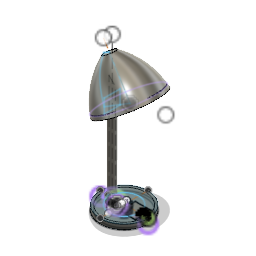
snailed_it v20 (Autodesk Fusion 360 design; units mm, degrees)
Autodesk Fusion 360 part; units mm, degrees
note: some values were not read from the file. Chosen so that the rebuilt part matches the saved one: which bodies a step acts on; a direction; which face or edge a step refers to. Set by a fixed rule: which sketch regions a step uses.
sketch "Sketch1" plane through (0, 0, 0) normal (0, 1, 0) x (1, 0, 0)
  circle A0 centre (0, 0) radius 150
  circle A1 centre (0, 0) radius 135
  dimension "d1" = 300
  dimension "d2" = 270
  constraint coincident A0.centre A1.centre
  measures "d1" diameter of A0
  measures "d2" diameter of A1
extrude "Extrude1" add sketch "Sketch1" along normal blind 30 makes body 1
sketch "Sketch2" plane through (0, 30, 0) normal (0, 1, 0) x (-1, 0, 0)
  circle A0 centre (0, 0) radius 135
  circle A1 centre (0, 0) radius 150
extrude "Extrude2" add sketch "Sketch2" along normal blind 2 separate body contours A0 | A1 makes body 2
sketch "Sketch3" plane through (0, 32, 0) normal (0, 1, 0) x (-1, 0, 0)
  circle A0 centre (0, 0) radius 150
  line L0 (0, 150) -> (0, 100) construction
  line L1 (0, 50) -> (0, -150) construction
  line L2 (150, 0) -> (-150, 0) construction
  circle A1 centre (75, 0) radius 25
  circle A2 centre (75, 0) radius 24
  point P0 (100, 0)
  point P1 (50, 0)
  dimension "d100" = 50
  dimension "d101" = 48
  dimension "d102" = 50
  dimension "d103" = 200
  constraint coincident A0 L0.start
  constraint coincident A0 L1.end
  constraint vertical L1
  constraint coincident A0 L2.start
  constraint coincident A0 L2.end
  constraint perpendicular L1 L2
  constraint coincident L2 A1.centre
  constraint concentric A1 A2
  constraint coincident L2 P0
  constraint coincident A1 P0
  constraint coincident A1 P1
  constraint coincident L2 P1
  measures "d100" diameter of A1
  measures "d101" diameter of A2
  measures "d102" distance of L2.start P0
  measures "d103" distance of L2.end P1
sketch "Sketch25" plane through (0, 0, 0) normal (0, 1, 0) x (1, 0, 0)
  circle A0 centre (-75, 0) radius 15
  point P0 (-75, 0)
  dimension "d142" = 30
  constraint coincident P0 A0.centre
  measures "d142" diameter of A0
extrude "Extrude4" cut sketch "Sketch25" along normal blind 130 bodies 2
extrude "Extrude3" add sketch "Sketch3" along normal blind 10 separate body contours A1 makes body 3
sketch "Sketch4" plane through (0, 32, 0) normal (0, 1, 0) x (-1, 0, 0)
  circle A0 centre (75, 0) radius 24
  circle A1 centre (75, 0) radius 23
  dimension "d104" = 48
  dimension "d105" = 46
  constraint concentric A0 A1
  measures "d104" diameter of A0
  measures "d105" diameter of A1
extrude "Extrude5" add sketch "Sketch4" along normal blind 700 separate body makes body 4
sketch "Sketch5" plane through (0, 30, 0) normal (0, 1, 0) x (-1, 0, 0)
  circle A0 centre (0, 0) radius 40
  circle A1 centre (0, 0) radius 91.8342
  dimension "d17" = 80
  constraint coincident A0.centre A1.centre
  constraint concentric A0 A1
  measures "d17" diameter of A0
sketch "Sketch6" plane through (0, 0, 0) normal (0, 0, 1) x (1, 0, 0)
  line L0 (150, 0) -> (-150, 0)
  line L1 (-75, 0) -> (0, 0) construction
  line L2 (-75, 0) -> (-75, 918.0902) construction
  line L3 (-55, 0) -> (-55, 645) construction
  line L4 (-95, 0) -> (-95, 685) construction
  line L5 (-95, 685) -> (-55, 645) construction
  point P0 (-75, 0)
  dimension "d106" = 75
  dimension "d108" = 20
  dimension "d109" = 20
  dimension "d110" = 685
  dimension "d112" = 45
  constraint perpendicular L1 L2
  constraint coincident L1.end origin
  constraint coincident L1 L3.start
  constraint coincident L0 L3.start
  constraint perpendicular L1 L3
  constraint coincident L0 L4.start
  constraint perpendicular L0 L4
  constraint coincident P0 L1.start
  measures "d106" distance of L1.end L1.start
  measures "d108" distance of L3.start P0
  measures "d109" distance of L4.start P0
  measures "d110" distance of L4.start L4.end
  measures "d112" angle of L4 L5
ref_plane "WorkPlane1" through (-75, 665, 0) normal (-0.707107, -0.707107, 0) x (0.707107, -0.707107, 0)
split "Split1" by plane through (-75, 665, 0) normal (-0.707107, -0.707107, 0) bodies 4 makes body 5 at (-66.9562, 448.9028, 22.6119)
delete_body "RemoveBody1" bodies 4
sketch "Sketch7" plane through (295, 295, 0) normal (-0.707107, -0.707107, 0) x (0.707107, -0.707107, 0)
  circle A0 centre (-523.2616, 0) radius 61
  point P0 (-523.2616, 0)
  dimension "d113" = 122
  constraint coincident P0 A0.centre
  measures "d113" diameter of A0
extrude "Extrude8" add sketch "Sketch7" against normal blind 2 separate body makes body 6
sketch "Sketch8" plane through (296.4142, 296.4142, 0) normal (0.707107, 0.707107, 0) x (0, 0, -1)
  circle A0 centre (0, 523.2616) radius 51
  circle A1 centre (0, 523.2616) radius 61
  point P0 (0, 523.2616)
  point P1 (0.1543, 462.2618)
  dimension "d32" = 102
  constraint coincident P0 A0.centre
  constraint coincident A1 P1
  measures "d32" diameter of A0
extrude "Extrude9" add sketch "Sketch8" along normal blind 6 separate body contours A0 makes body 7
sketch "Sketch9" plane through (296.4142, 296.4142, 0) normal (0.707107, 0.707107, 0) x (0, 0, -1)
  circle A0 centre (0, 523.2616) radius 61
  circle A1 centre (0, 523.2616) radius 52
  circle A2 centre (0, 523.2616) radius 61
  line L0 (-26.4064, 478.4654) -> (-31.9044, 471.2701)
  line L1 (26.4064, 478.4654) -> (31.9044, 471.2701)
  point P0 (0, 523.2616)
  dimension "d35" = 122
  dimension "d36" = 104
  constraint concentric A0 A1
  constraint coincident P0 A0.centre
  constraint coincident A1 L0.start
  constraint coincident A2 L0.end
  constraint coincident A1 L1.start
  constraint coincident A2 L1.end
  constraint coincident A0 L1.end
  constraint equal L0 L1
  measures "d35" diameter of A0
  measures "d36" diameter of A1
extrude "Extrude10" add sketch "Sketch9" along normal blind 6 separate body contours A0 A1 A2 L0 L1 picked at (-34.6439, 476.9097) makes body 8
sketch "Sketch10" plane through (300.6569, 300.6569, 0) normal (0.707107, 0.707107, 0) x (0, 0, -1)
  circle A0 centre (0, 523.2616) radius 61
  line L0 (-61, 523.2616) -> (61, 523.2616) construction
  line L1 (0.0652, 584.2615) -> (0.0652, 462.2616) construction
  line L2 (-57.2713, 544.2615) -> (57.2713, 544.2615)
  line L3 (-57.2713, 502.2616) -> (57.2713, 502.2616)
  line L4 (-45.1664, 482.2616) -> (45.1664, 482.2616)
  arc A1 (26.4064, 478.4654) -> (-26.4064, 478.4654) centre (0, 523.2616) ccw
  line L5 (26.4064, 478.4654) -> (31.9044, 471.2701)
  arc A2 (31.9044, 471.2701) -> (-31.9044, 471.2701) centre (0, 523.2616) ccw
  line L6 (-31.9044, 471.2701) -> (-26.4064, 478.4654)
  point P0 (0, 544.2615)
  point P1 (0, 502.2616)
  point P2 (0, 482.2616)
  dimension "d39" = 122
  dimension "d66" = 40
  dimension "d67" = 20
  dimension "d68" = 20
  constraint coincident A0 L0.start
  constraint coincident A0 L0.end
  constraint coincident A0.centre L0
  constraint coincident A0 L1.start
  constraint coincident A0 L1.end
  constraint vertical L1
  constraint coincident A0 L2.start
  constraint coincident A0 L2.end
  constraint parallel L0 L2
  constraint coincident A0 L3.start
  constraint coincident A0 L3.end
  constraint parallel L0 L3
  constraint coincident A0 L4.start
  constraint coincident A0 L4.end
  constraint parallel L3 L4
  constraint perpendicular L1 L2
  constraint midpoint L2 P0
  constraint midpoint L3 P1
  constraint midpoint L4 P2
  measures "d39" diameter of A0
  measures "d66" vertical distance of L1.start P0
  measures "d67" distance of P1 P2
  measures "d68" vertical distance of L1.end P2
extrude "Extrude12" add sketch "Sketch10" along normal blind 2 separate body contours A0 L2 A1 A2 | A0 L3 L4 A1 A2 | L2 A1 | L3 L4 A1 | A0 L3 L4 A1 A2 makes body 9 at (-103.1191, 704.4328, 16.3292) makes body 10 at (-46.512, 647.8258, -17.4627)
sketch "Sketch11" plane through (300.6569, 300.6569, 0) normal (0.707107, 0.707107, 0) x (0, 0, -1)
  circle A0 centre (0, 523.2616) radius 51
  circle A1 centre (0, 523.2616) radius 51 construction
  line L0 (-0.0016, 574.2616) -> (-0.0016, 472.2616) construction
  line L1 (-51, 523.2616) -> (51, 523.2616) construction
  line L2 (-50.3686, 531.2616) -> (-50.3686, 515.2616)
  point P0 (-50.3686, 523.2616)
  dimension "d76" = 16
  constraint coincident A0.centre A1.centre
  constraint coincident A1 L0.start
  constraint coincident A0 L0.end
  constraint vertical L0
  constraint coincident A1 L0.end
  constraint coincident A1 L1.start
  constraint coincident A0 L1.end
  constraint perpendicular L0 L1
  constraint coincident A0 L2.start
  constraint coincident A0 L2.end
  constraint perpendicular L1 L2
  constraint midpoint L2 P0
  measures "d76" distance of L2.start L2.end
ref_plane "WorkPlane3" through (-69.3449, 670.6586, 0.0016) normal (0, 0, 1) x (0.707107, -0.707107, 0)
sketch "Sketch16" plane through (0, 0, 0.0016) normal (0, 0, 1) x (0.642788, 0.766044, 0)
  line L0 (469.8775, 492.1819) -> (468.483, 476.2428)
  circle A0 centre (535.9253, 478.3729) radius 8
  line L1 (469.8775, 492.1819) -> (536.6226, 486.3425)
  line L2 (468.483, 476.2428) -> (535.228, 470.4034)
  line L3 (469.1803, 484.2124) -> (535.9253, 478.3729)
  line L4 (535.9253, 478.3729) -> (543.8949, 477.6757)
  line L5 (464.6489, 432.4188) -> (474.4968, 544.9803)
  point P0 (469.8775, 492.1819)
  point P1 (468.483, 476.2428)
  point P2 (469.1803, 484.2124)
  point P3 (464.6489, 432.4188)
  dimension "d78" = 16
  dimension "d79" = 16
  dimension "d80" = 75
  constraint coincident P0 L0.start
  constraint coincident P1 L0.end
  constraint coincident P2 L0
  constraint coincident A0 L1.end
  constraint parallel L1 L2
  constraint coincident P2 L3.start
  constraint coincident A0.centre L3.end
  constraint coincident A0 L4.end
  constraint parallel L3 L4
  constraint coincident A0 L2.end
  constraint coincident P1 L5
  measures "d78" distance of P0 L0.end
  measures "d79" diameter of A0
  measures "d80" distance of P2 L4.end
extrude "Extrude14" add sketch "Sketch16" along normal blind 4 from surface at 46 separate body makes body 11
mirror "Mirror2" about plane through (-69.3449, 670.6586, 0.0016) normal (0, 0, 1) of bodies 11 makes body 12
extrude "Extrude15" cut sketch "Sketch9" against normal blind 2 contours A0 A1 A2 L0 L1 picked at (27.5941, 472.3736) bodies 6
sketch "Sketch21" plane through (0, 0, 0) normal (0, 0, 1) x (1, 0, 0)
  line L0 (-83.2468, 732.5263) -> (-2.3286, 591.0298) construction
  line L1 (-2.3286, 591.0298) -> (77.5344, 636.7015) construction
  line L2 (-83.2468, 732.5263) -> (-3.3838, 778.1979) construction
  line L3 (-3.3838, 778.1979) -> (77.5344, 636.7015) construction
  line L4 (-43.3153, 755.3621) -> (37.6029, 613.8657) construction
  line L5 (-61.9003, 695.199) -> (17.9627, 740.8706) construction
  arc A0 (-16.312, 712.3779) -> (-27.6256, 723.6917) centre (-21.9688, 718.0348) ccw
  line L6 (-21.9688, 718.0348) -> (-69.3449, 670.6586)
  line L7 (-63.6881, 665.0018) -> (-16.312, 712.3779)
  line L8 (-75.0018, 676.3155) -> (-63.6881, 665.0018)
  line L9 (-109.65, 702.4785) -> (-83.2468, 732.5263) construction
  line L10 (-37.5251, 630.3536) -> (-109.65, 702.4785)
  point P0 (-21.9688, 718.0348)
  dimension "d122" = 163
  dimension "d143" = 92
  dimension "d144" = 43
  dimension "d148" = 40
  constraint perpendicular L0 L1
  constraint parallel L1 L2
  constraint parallel L0 L3
  constraint midpoint L2 L4.start
  constraint midpoint L1 L4.end
  constraint coincident L0 L5.start
  constraint coincident L3 L5.end
  constraint perpendicular L3 L5
  constraint midpoint L5 P0
  constraint coincident P0 A0.centre
  constraint parallel L6 L7
  constraint coincident L6.end L8
  constraint coincident L9.start L10.end
  measures "d122" distance of L0.end L0.start
  measures "d143" distance of L0.end L1.end
  measures "d144" distance of L2 L5
  measures "d148" distance of L0.start L9.start
ref_plane "WorkPlane4" through (37.6029, 613.8657, 0) normal (0.496431, -0.868076, 0) x (0.868076, 0.496431, 0)
sketch "Sketch22" plane through (-255.2722, 446.3778, 0) normal (0.496431, -0.868076, 0) x (0.868076, 0.496431, 0)
  circle A0 centre (337.3841, 0) radius 46
  point P0 (291.3841, 0)
  point P1 (383.3841, 0)
  point P2 (337.3841, 0)
  dimension "d117" = 92
  constraint coincident P2 A0.centre
  measures "d117" diameter of A0
extrude "Extrude16" add sketch "Sketch22" against normal blind 163 separate body makes body 13
sketch "Sketch23" plane through (0, 0, 0) normal (0, 0, 1) x (1, 0, 0)
  line L0 (37.7571, 600.1582) -> (-129.6519, 872.1977) construction
  line L1 (36.9149, 599.6443) -> (-94.1095, 812.5588)
  line L2 (36.9149, 599.6443) -> (-124.8983, 500.0626)
  arc A0 (-126.5916, 792.8111) -> (-124.8983, 500.0626) centre (261.3334, 648.6758) ccw
  line L3 (-126.5916, 792.8111) -> (-94.1095, 812.5588)
  point P0 (37.7571, 600.1582)
  dimension "d154" = 250
  dimension "d160" = 380
  dimension "d161" = 78
  constraint coincident P0 L0.start
  constraint coincident L1.start L2.start
  measures "d154" distance of L1.start L1.end
revolve "Revolve1" add sketch "Sketch23" angle 360 about axis through (37.7571, 600.1582, 0) along (-0.524097, 0.851658, 0) separate body makes body 14
sketch "Sketch24" plane through (0, 32, 0) normal (0, 1, 0) x (-1, 0, 0)
  circle A0 centre (0, 0) radius 150
  circle A1 centre (15, 10) radius 5
  circle A2 centre (15, 30) radius 5
  circle A3 centre (15, -10) radius 5
  circle A4 centre (15, -30) radius 5
  line L0 (-20, 50) -> (-120, 50)
  line L1 (-120, 50) -> (-120, -50)
  line L2 (-120, -50) -> (-20, -50)
  line L3 (-20, -50) -> (-20, 50)
  circle A5 centre (75, 0) radius 15
  point P0 (50, 0)
  point P1 (15, 0)
  point P2 (-150, 0)
  point P3 (-120, 0)
  dimension "d124" = 10
  dimension "d128" = 10
  dimension "d129" = 10
  dimension "d130" = 10
  dimension "d137" = 100
  dimension "d138" = 100
  dimension "d139" = 30
  constraint horizontal L0
  constraint vertical L1
  constraint horizontal L2
  constraint vertical L3
  constraint coincident A0 P2
  constraint midpoint L1 P3
  measures "d124" diameter of A1
  measures "d128" diameter of A2
  measures "d129" diameter of A3
  measures "d130" diameter of A4
  measures "d137" distance of L0.start L0.end
  measures "d138" distance of L0.start L2.end
  measures "d139" distance of P2 P3
ref_plane "WorkPlane5" through (-15, 0, 0) normal (1, 0, 0) x (0, 1, 0)
extrude "Extrude22" cut sketch "Sketch24" against normal through all contours A1 | A2 | A3 | A4 bodies 2
sketch "Sketch26" plane through (-15, 0, 0) normal (1, 0, 0) x (0, 0, -1)
  line L0 (-25, 32) -> (-35, 32)
  line L1 (-34.1863, 24) -> (-34.1863, 39.7946)
  line L2 (-34.1863, 39.7946) -> (-25.8137, 39.7946)
  line L3 (-25.8137, 39.7946) -> (-25.8137, 23.5453)
  line L4 (-25.8137, 23.5453) -> (-21.2835, 23.5453)
  line L5 (-21.2835, 23.5453) -> (-21.2835, 20.1946)
  line L6 (-21.2835, 20.1946) -> (-38.7165, 20.1946)
  line L7 (-38.7165, 20.1946) -> (-38.7165, 24)
  line L8 (-38.7165, 24) -> (-34.1863, 24)
  line L9 (-30, 39.7946) -> (-30, 20.1946)
  point P0 (-30, 32)
  constraint perpendicular L1 L2
  constraint perpendicular L0 L3
  constraint perpendicular L3 L4
  constraint perpendicular L0 L5
  constraint perpendicular L5 L6
  constraint perpendicular L0 L7
  constraint midpoint L2 L9.start
  constraint coincident L6 L9.end
  constraint perpendicular L6 L9
  constraint coincident L1.start L8.end
  constraint vertical L1
  constraint horizontal L8
  constraint equal L4 L8
  constraint midpoint L0 P0
  constraint coincident L9 P0
sketch "Sketch27" plane through (-15, 0, 0) normal (1, 0, 0) x (0, 0, -1)
  line L0 (-34.1863, 24) -> (-34.1863, 39.7946)
  line L1 (-34.1863, 39.7946) -> (-25.8137, 39.7946)
  line L2 (-25.8137, 39.7946) -> (-25.8137, 23.5453)
  circle A0 centre (-30, 44.5846) radius 3.537
  arc A1 (-20.3559, 34.0749) -> (-27.4915, 47.0782) centre (-46.4897, 28.1933) ccw
  line L3 (-30, 48.1216) -> (-30, 40.4192)
  line L4 (-30, 40.4192) -> (-25.3401, 40.4192)
  line L5 (-25.3401, 40.4192) -> (-25.3401, 34.0749)
  line L6 (-25.3401, 34.0749) -> (-20.3559, 34.0749)
  point P0 (-30, 39.7946)
  constraint tangent A0 A1
  constraint coincident A0 A1.end
  constraint coincident A0 L3.start
  constraint vertical L3
  constraint coincident L3 L4.start
  constraint perpendicular L3 L4
  constraint perpendicular L4 L5
  constraint coincident A0.centre L3
  constraint coincident L3.end L4.start
  constraint vertical L3.end P0
  constraint horizontal L6
revolve "Revolve2" add sketch "Sketch26" angle 360 about axis through (-15, 39.7946, 30) along (0, -1, 0) separate body contours L0 L3 L4 L5 L6 L9 | L0 L2 L3 L9 makes body 15
revolve "Revolve3" add sketch "Sketch27" angle 360 about axis through (-15, 48.1216, 30) along (0, -1, 0) separate body contours A0 L3 | A0 A1 L3 L4 L5 L6 picked at (-28.6425, 45.7054) makes body 16
extrude "Extrude17" add sketch "Sketch24" along normal blind 5 contours A1 bodies 2
extrude "Extrude18" add sketch "Sketch24" along normal blind 5 contours A2 bodies 2
extrude "Extrude19" add sketch "Sketch24" along normal blind 5 separate body contours A3 makes body 17
extrude "Extrude20" add sketch "Sketch24" along normal blind 5 contours A4 bodies 2
extrude "Extrude21" add sketch "Sketch24" along normal blind 2 separate body contours L0 L1 L2 L3 makes body 18
shell "Shell1" thickness 3 removed faces 1 at (84.0441, 628.6435, -138.4809) on bodies 14
ref_plane "WorkPlane6" through (91.1901, 633.0422, 72.6429) normal (-0.524087, 0.851665, 0.000015) x (-0.644537, -0.396638, 0.653644)
ref_plane "WorkPlane7" through (80.7083, 650.0755, 72.6432) normal (-0.524087, 0.851665, 0.000015) x (-0.644537, -0.396638, 0.653644)
sketch "Sketch30" plane through (-267.9914, 435.4984, 0.0075) normal (-0.524087, 0.851665, 0.000015) x (0.000008, -0.000013, 1)
  spline S0 degree 3 poles (138.9862, 466.7387) (142.6901, 462.4502) (146.3638, 457.7892) (153.3622, 447.909) (156.6868, 442.6898) (162.7844, 431.9415) (165.5588, 426.4101) (170.4491, 415.334) (172.5653, 409.7894) (176.127, 399.0306) (177.7373, 393.3184) (180.422, 381.5121) (181.4962, 375.418) (183.0165, 363.1544) (183.4628, 356.9824) (183.7423, 344.878) (183.5755, 338.9455) (182.7488, 327.6427) (182.0506, 321.7492) (180.0128, 309.8142) (178.6731, 303.7728) (175.3846, 291.861) (173.4351, 285.988) (169.0611, 274.6981) (166.6368, 269.281) (161.5476, 259.155) (158.6472, 253.9773) (152.1972, 243.7306) (148.6476, 238.6618) (141.0509, 228.9152) (137.0023, 224.2353) (128.6408, 215.4787) (124.328, 211.4017) (115.7512, 203.994) (111.0901, 200.3204) (101.2099, 193.3221) (95.9907, 189.9975) (85.2425, 183.8999) (79.7112, 181.1256) (68.6351, 176.2353) (63.0905, 174.1192) (52.3317, 170.5576) (46.6196, 168.9473) (34.8134, 166.2626) (28.7193, 165.1884) (16.4558, 163.6682) (10.2838, 163.2218) (-1.8206, 162.9424) (-7.753, 163.1091) (-19.0557, 163.9359) (-24.9492, 164.6341) (-36.8841, 166.6718) (-42.9254, 168.0115) (-54.8372, 171.3) (-60.7101, 173.2495) (-72, 177.6234) (-77.417, 180.0477) (-87.543, 185.1368) (-92.7207, 188.0372) (-102.9673, 194.4871) (-108.0361, 198.0367) (-117.7827, 205.6333) (-122.4626, 209.6819) (-131.2192, 218.0433) (-135.2962, 222.356) (-142.7038, 230.9328) (-146.3775, 235.5939) (-153.3759, 245.474) (-156.7004, 250.6931) (-162.798, 261.4413) (-165.5724, 266.9726) (-170.4627, 278.0486) (-172.5789, 283.5932) (-176.1405, 294.3519) (-177.7508, 300.064) (-180.4356, 311.8701) (-181.5098, 317.9643) (-183.0301, 330.2277) (-183.4766, 336.3997) (-183.7561, 348.504) (-183.5894, 354.4364) (-182.7627, 365.7392) (-182.0645, 371.6327) (-180.0269, 383.5676) (-178.6872, 389.6089) (-175.3988, 401.5207) (-173.4494, 407.3937) (-169.0755, 418.6836) (-166.6512, 424.1007) (-161.5621, 434.2267) (-158.6617, 439.4045) (-152.2119, 449.6511) (-148.6623, 454.7199) (-141.0658, 464.4666) (-137.0172, 469.1465) (-128.6558, 477.9033) (-124.343, 481.9802) (-115.7663, 489.388) (-111.1052, 493.0617) (-101.2251, 500.0601) (-96.0059, 503.3847) (-85.2578, 509.4824) (-79.7264, 512.2568) (-68.6504, 517.1472) (-63.1057, 519.2634) (-52.347, 522.8251) (-46.6349, 524.4354) (-34.8286, 527.1202) (-28.7344, 528.1944) (-16.4709, 529.7148) (-10.2989, 530.1612) (1.8055, 530.4407) (7.7379, 530.274) (19.0408, 529.4474) (24.9343, 528.7492) (36.8693, 526.7115) (42.9107, 525.3719) (54.8225, 522.0834) (60.6956, 520.1339) (71.9856, 515.76) (77.4026, 513.3357) (87.5287, 508.2466) (92.7065, 505.3461) (102.9532, 498.8963) (108.022, 495.3466) (117.7687, 487.75) (122.4486, 483.7014) (131.2054, 475.3399) (135.2823, 471.0271) (138.9862, 466.7387) knots 0 0 0 0 1.69995263 1.69995263 3.39990527 3.39990527 5.0998579 5.0998579 6.79981053 6.79981053 8.49976197 8.49976197 10.19971341 10.19971341 11.89966485 11.89966485 13.59961629 13.59961629 15.29956553 15.29956553 16.99951477 16.99951477 18.69946401 18.69946401 20.39941324 20.39941324 22.0993596 22.0993596 23.79930596 23.79930596 25.49925232 25.49925232 27.19919868 27.19919868 28.89914192 28.89914192 30.59908516 30.59908516 32.29902841 32.29902841 33.99897165 33.99897165 35.69891202 35.69891202 37.39885238 37.39885238 39.09879274 39.09879274 40.79873311 40.79873311 42.49867127 42.49867127 44.19860943 44.19860943 45.89854759 45.89854759 47.59848575 47.59848575 49.29842272 49.29842272 50.99835969 50.99835969 52.69829666 52.69829666 54.39823363 54.39823363 56.09817059 56.09817059 57.79810756 57.79810756 59.49804453 59.49804453 61.1979815 61.1979815 62.89791966 62.89791966 64.59785782 64.59785782 66.29779598 66.29779598 67.99773414 67.99773414 69.69767451 69.69767451 71.39761487 71.39761487 73.09755524 73.09755524 74.7974956 74.7974956 76.49743884 76.49743884 78.19738209 78.19738209 79.89732533 79.89732533 81.59726857 81.59726857 83.29721493 83.29721493 84.99716129 84.99716129 86.69710765 86.69710765 88.39705401 88.39705401 90.09700325 90.09700325 91.79695248 91.79695248 93.49690172 93.49690172 95.19685096 95.19685096 96.8968024 96.8968024 98.59675384 98.59675384 100.29670528 100.29670528 101.99665672 101.99665672 103.69660935 103.69660935 105.39656199 105.39656199 107.09651462 107.09651462 108.79646725 108.79646725 108.79646725 108.79646725
extrude "Extrude24" add sketch "Sketch30" along normal blind 3 separate body makes body 19
ref_plane "WorkPlane8" through (-75, 0, 0) normal (1, 0, 0) x (0, 1, 0)
sketch "Sketch31" plane through (-75, 0, 0) normal (1, 0, 0) x (0, 0, -1)
  line L0 (49.1072, 597.6175) -> (-50, 597.6175)
  line L1 (-50, 597.6175) -> (-50, 510)
  line L2 (-50, 510) -> (49.1072, 510)
  line L3 (49.1072, 510) -> (49.1072, 597.6175)
  constraint horizontal L0
  constraint vertical L1
  constraint horizontal L2
  constraint vertical L3
extrude "Extrude25" add sketch "Sketch31" along normal up to surface end surface at (-141.0466, 622.6662, -59.2187) on bodies 14 bodies 5 14
extrude "Extrude26" add sketch "Sketch31" along normal blind 30 separate body makes body 20
hidden bodies 9
equation "tubes = 2 mm"
equation "d54 = 51 mm - 5 mm"
equation "d101 = 50 mm - tubes"
equation "d104 = 50 mm - tubes"
equation "d105 = 50 mm - 2 * tubes"
